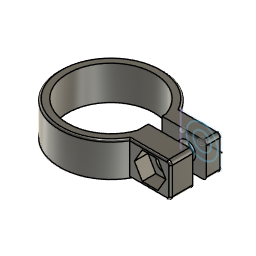
3D Shaft Collar v7 (Autodesk Fusion 360 design; units mm, degrees)
Autodesk Fusion 360 part; units mm, degrees
sketch "Sketch1" plane through (0, 0, 0) normal (0, 0, 1) x (1, 0, 0)
  circle A0 centre (0, 0) radius 12.7
  circle A1 centre (0, 0) radius 15
  dimension "d1" = 25.4
  dimension "d27" = 30
  constraint coincident A0.centre A1.centre
  constraint concentric A0 A1
  measures "d1" diameter of A0
  measures "d27" diameter of A1
extrude "Extrude1" add sketch "Sketch1" along normal blind 10
ref_plane "WorkPlane1" through (15, 0, 6.109) normal (1, 0, 0) x (0, -1, 0)
sketch "Sketch2" plane through (15, 0, 0) normal (1, 0, 0) x (0, 1, 0)
  line L0 (0, 10) -> (0, 0)
  line L1 (7.5, 10) -> (-7.5, 10)
  line L2 (-7.5, 10) -> (-7.5, 0)
  line L3 (-7.5, 0) -> (7.5, 0)
  line L4 (7.5, 0) -> (7.5, 10)
  line L5 (7.5, 10) -> (-7.5, 0) construction
  line L6 (-7.5, 10) -> (7.5, 0) construction
  point P0 (0, 5)
  dimension "d5" = 15
  dimension "d6" = 10
  constraint coincident L0.end origin
  constraint vertical L0
  constraint horizontal L1
  constraint perpendicular L1 L2
  constraint parallel L1 L3
  constraint parallel L2 L4
  constraint coincident L5 P0
  constraint coincident L6 P0
  constraint midpoint L0 P0
  measures "d5" distance of L2.end L3.end
  measures "d6" distance of L1.end L2.end
extrude "Extrude2" add sketch "Sketch2" against normal blind 3
extrude "Extrude3" add 1 faces at (15, -2.5, 6.6667) along direction (1, 0, 0) blind 10
sketch "Sketch3" plane through (0, -7.5, 0) normal (0, -1, 0) x (-1, 0, 0)
  line L0 (-12.9904, 0) -> (-25, 0)
  line L1 (-25, 0) -> (-25, -10)
  line L2 (-25, -10) -> (-12.9904, -10)
  line L3 (-12.9904, -10) -> (-12.9904, 0)
  line L4 (-18.9952, -10) -> (-18.9952, 0)
  line L5 (-16.6858, -9) -> (-14.3764, -5)
  line L6 (-14.3764, -5) -> (-16.6858, -1)
  line L7 (-16.6858, -1) -> (-21.3046, -1)
  line L8 (-21.3046, -1) -> (-23.614, -5)
  line L9 (-23.614, -5) -> (-21.3046, -9)
  line L10 (-21.3046, -9) -> (-16.6858, -9)
  point P0 (-18.9952, -5)
  dimension "d28" = 4
  constraint midpoint L2 L4.start
  constraint midpoint L0 L4.end
  constraint midpoint L4 P0
  measures "d28" distance of P0 L10
extrude "Extrude4" cut sketch "Sketch3" against normal blind 4 contours L4 L5 L6 L7 L10 | L4 L7 L8 L9 L10
sketch "Sketch4" plane through (0, 7.5, 0) normal (0, 1, 0) x (1, 0, 0)
  line L0 (12.9904, -10) -> (25, -10)
  line L1 (25, -10) -> (25, 0)
  line L2 (25, 0) -> (12.9904, 0)
  line L3 (25, -5) -> (13.5185, -5)
  circle A0 centre (19.2593, -5) radius 2.6
  circle A1 centre (19.2593, -5) radius 4.6
  line L4 (12.9904, 0) -> (12.9904, -10)
  dimension "d14" = 5.2
  dimension "d15" = 9.2
  constraint midpoint L1 L3.start
  constraint midpoint L3 A0.centre
  constraint concentric A0 A1
  constraint horizontal L3
  measures "d14" diameter of A0
  measures "d15" diameter of A1
extrude "Extrude5" cut sketch "Sketch4" against normal blind 1.55 contours L3 A0 A1 | L3 A0 A1 | L3 A0 | L3 A0
extrude "Extrude6" cut sketch "Sketch4" against normal blind 16 contours L3 A0 | L3 A0
ref_plane "WorkPlane2" through (18.9952, 1, 5) normal (0, 1, 0) x (1, 0, 0)
sketch "Sketch5" plane through (0, 1, 0) normal (0, 1, 0) x (1, 0, 0)
  line L0 (9, 4) -> (34, 4)
  line L1 (34, 4) -> (34, -16)
  line L2 (34, -16) -> (9, -16)
  line L3 (9, -16) -> (9, 4)
  constraint horizontal L0
  constraint vertical L1
  constraint horizontal L2
  constraint vertical L3
extrude "Extrude7" cut sketch "Sketch5" along normal mid plane 4
fillet "Fillet1" radius 1 4 edges at (25, 5.25, 0) (25, -4.25, 0) (25, 5.25, 10) (25, -4.25, 10)
fillet "Fillet2" radius 0.5 11 edges at (18.4952, 7.5, 10) (24.7071, 7.5, 9.7071) (25, 7.5, 5) (24.7071, 7.5, 0.2929) (18.4952, 7.5, 0) (18.4952, -7.5, 10) (24.7071, -7.5, 9.7071) (25, -7.5, 5) (24.7071, -7.5, 0.2929) (18.4952, -7.5, 0) (-15, 0, 10)
